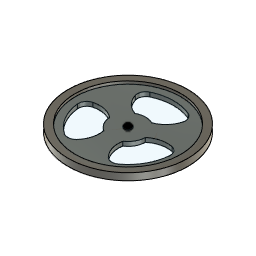
integerater v4 (Autodesk Fusion 360 archive; units mm, degrees)
design "wheel_edited"
Autodesk Fusion 360 part; units mm, degrees
note: some values were not read from the file. Chosen so that the rebuilt part matches the saved one: which bodies a step acts on; which face or edge a step refers to. Set by a fixed rule: which sketch regions a step uses.
sketch "Sketch1" plane through (0, 0, 0) normal (0, 0, 1) x (1, 0, 0)
  circle A0 centre (0, 0) radius 12.5
  circle A1 centre (0, 0) radius 37.5
  arc A2 (-17.0167, 22.1752) -> (-6.0591, 10.9333) centre (-0.423, 27.3882) ccw
  arc A3 (5.7186, 11.1152) -> (16.3238, 22.6902) centre (-0.423, 27.3882) ccw
  arc A4 (-12.4853, -0.6052) -> (-27.8122, 2.7918) centre (-23.5074, -14.0604) ccw
  arc A5 (-10.696, -25.8245) -> (-6.439, -10.714) centre (-23.5074, -14.0604) ccw
  arc A6 (27.7127, 3.6493) -> (12.4981, -0.2194) centre (23.9303, -13.3278) ccw
  arc A7 (6.7668, -10.51) -> (11.4883, -25.4819) centre (23.9303, -13.3278) ccw
  arc A8 (-32.288, -3.7057) -> (-18.5377, -26.6946) centre (0, 0) ccw
  arc A9 (19.3532, -26.1094) -> (32.3871, -2.7068) centre (0, 0) ccw
  arc A10 (12.9348, 29.8151) -> (-13.8494, 29.4015) centre (0, 0) ccw
  arc A11 (-27.8122, 2.7918) -> (-32.288, -3.7057) centre (-26.3272, -3.0216) ccw
  arc A12 (-18.5377, -26.6946) -> (-10.696, -25.8245) centre (-15.1154, -21.7664) ccw
  arc A13 (11.4883, -25.4819) -> (19.3532, -26.1094) centre (15.7803, -21.2892) ccw
  arc A14 (32.3871, -2.7068) -> (27.7127, 3.6493) centre (26.4079, -2.2071) ccw
  arc A15 (16.3238, 22.6902) -> (12.9348, 29.8151) centre (10.5468, 24.3108) ccw
  arc A16 (-13.8494, 29.4015) -> (-17.0167, 22.1752) centre (-11.2925, 23.9735) ccw
  dimension "d1" = 65
  dimension "d2" = 25
  dimension "d3" = 75
  dimension "d6" = 6
  dimension "d7" = 6
  dimension "d8" = 6
  constraint coincident A0.centre A1.centre
  constraint coincident A0 A2.end
  constraint coincident A0 A3.start
  constraint concentric A2 A3
  constraint coincident A0 A5.end
  constraint coincident A0 A4.start
  constraint concentric A4 A5
  constraint coincident A0 A6.end
  constraint coincident A0 A7.start
  constraint concentric A6 A7
  constraint concentric A8 A9
  constraint concentric A9 A10
  constraint tangent A4 A11
  constraint tangent A8 A11
  constraint tangent A8 A12
  constraint tangent A5 A12
  constraint tangent A7 A13
  constraint tangent A9 A13
  constraint equal A12 A13
  constraint tangent A9 A14
  constraint tangent A6 A14
  constraint equal A12 A14
  constraint tangent A3 A15
  constraint tangent A10 A15
  constraint equal A12 A15
  constraint tangent A2 A16
  constraint tangent A10 A16
  measures "d1" diameter of A8
  measures "d2" diameter of A0
  measures "d3" diameter of A1
  measures "d6" radius of A11
  measures "d7" radius of A12
  measures "d8" radius of A16
extrude "Extrude1" add sketch "Sketch1" along normal blind 3 contours A0 | A1
sketch "Sketch2" plane through (0, 0, 3) normal (0, 0, 1) x (-1, 0, 0)
  arc A0 (12.4853, 0.6052) -> (27.8122, -2.7918) centre (23.5074, 14.0604) ccw
  arc A1 (12.4853, 0.6052) -> (6.439, 10.714) centre (0, 0) ccw
  arc A2 (10.696, 25.8245) -> (6.439, 10.714) centre (23.5074, 14.0604) ccw
  arc A3 (18.5377, 26.6946) -> (10.696, 25.8245) centre (15.1154, 21.7664) ccw
  arc A4 (32.288, 3.7057) -> (18.5377, 26.6946) centre (0, 0) ccw
  arc A5 (27.8122, -2.7918) -> (32.288, 3.7057) centre (26.3272, 3.0216) ccw
  arc A6 (-6.7668, 10.51) -> (-11.4883, 25.4819) centre (-23.9303, 13.3278) ccw
  arc A7 (-6.7668, 10.51) -> (-12.4981, 0.2194) centre (0, 0) ccw
  arc A8 (-27.7127, -3.6493) -> (-12.4981, 0.2194) centre (-23.9303, 13.3278) ccw
  arc A9 (-32.3871, 2.7068) -> (-27.7127, -3.6493) centre (-26.4079, 2.2071) ccw
  arc A10 (-19.3532, 26.1094) -> (-32.3871, 2.7068) centre (0, 0) ccw
  arc A11 (-11.4883, 25.4819) -> (-19.3532, 26.1094) centre (-15.7803, 21.2892) ccw
  arc A12 (-5.7186, -11.1152) -> (-16.3238, -22.6902) centre (0.423, -27.3882) ccw
  arc A13 (-5.7186, -11.1152) -> (6.0591, -10.9333) centre (0, 0) ccw
  arc A14 (17.0167, -22.1752) -> (6.0591, -10.9333) centre (0.423, -27.3882) ccw
  arc A15 (13.8494, -29.4015) -> (17.0167, -22.1752) centre (11.2925, -23.9735) ccw
  arc A16 (-12.9348, -29.8151) -> (13.8494, -29.4015) centre (0, 0) ccw
  arc A17 (-16.3238, -22.6902) -> (-12.9348, -29.8151) centre (-10.5468, -24.3108) ccw
  circle A18 centre (0, 0) radius 37.5
  circle A19 centre (0, 0) radius 2.3
  line L0 (-1.5578, 1.6921) -> (-1.5578, -1.6921)
  line L1 (1.5578, -1.6921) -> (1.5578, 1.6921)
  line L2 (1.5578, 1.6921) -> (-1.5578, -1.6921) construction
  line L3 (-1.5578, 1.6921) -> (1.5578, -1.6921) construction
  dimension "d11" = 4.6
  dimension "d42" = 3.3843
  constraint concentric A1 A19
  constraint parallel L0 L1
  constraint coincident L2 A1.centre
  constraint coincident L3 A1.centre
  constraint coincident A1.centre A4.centre
  constraint coincident A19 L0.start
  measures "d11" diameter of A19
  measures "d42" distance of L0.start L0.end
extrude "Extrude2" add sketch "Sketch2" along normal blind 1.5 contours A19 L1 | A19 L0 L1 | A19 L0
sketch "Sketch3" plane through (0, 0, 0) normal (0, 0, 1) x (1, 0, 0)
  circle A0 centre (0, 0) radius 42.5
  spline S0 degree 2 poles (3.0979, -42.3869) (0, -46) (-3.0574, -42.3899) knots 0 0 0 0.819978 0.819978 0.819978 weights 1 3 1
  spline S1 degree 2 poles (8.386, -41.6644) (5.7653, -45.6373) (2.2796, -42.4388) knots 0 0 0 0.819978 0.819978 0.819978 weights 1 3 1
  spline S2 degree 2 poles (13.5418, -40.2849) (11.4397, -44.5548) (7.5806, -41.8185) knots 0 0 0 0.819978 0.819978 0.819978 weights 1 3 1
  spline S3 degree 2 poles (18.484, -38.27) (16.9337, -42.7697) (12.762, -40.5386) knots 0 0 0 0.819978 0.819978 0.819978 weights 1 3 1
  spline S4 degree 2 poles (23.1348, -35.6515) (22.1607, -40.3101) (17.7422, -38.6195) knots 0 0 0 0.819978 0.819978 0.819978 weights 1 3 1
  spline S5 degree 2 poles (27.4207, -32.4708) (27.0381, -37.2148) (22.4426, -36.0912) knots 0 0 0 0.819978 0.819978 0.819978 weights 1 3 1
  spline S6 degree 2 poles (31.2741, -28.7781) (31.4892, -33.5326) (26.7891, -32.9938) knots 0 0 0 0.819978 0.819978 0.819978 weights 1 3 1
  spline S7 degree 2 poles (34.6344, -24.6315) (35.4436, -29.3215) (30.7131, -29.3761) knots 0 0 0 0.819978 0.819978 0.819978 weights 1 3 1
  spline S8 degree 2 poles (37.4484, -20.0964) (38.8391, -24.648) (34.1527, -25.2951) knots 0 0 0 0.819978 0.819978 0.819978 weights 1 3 1
  spline S9 degree 2 poles (39.6719, -15.2444) (41.622, -19.5858) (37.0537, -20.8152) knots 0 0 0 0.819978 0.819978 0.819978 weights 1 3 1
  spline S10 degree 2 poles (41.2697, -10.152) (43.7486, -14.2148) (39.3704, -16.007) knots 0 0 0 0.819978 0.819978 0.819978 weights 1 3 1
  spline S11 degree 2 poles (42.2166, -4.8995) (45.1852, -8.6195) (41.0661, -10.9463) knots 0 0 0 0.819978 0.819978 0.819978 weights 1 3 1
  spline S12 degree 2 poles (42.4978, 0.4303) (45.9092, -2.8884) (42.1143, -5.7131) knots 0 0 0 0.819978 0.819978 0.819978 weights 1 3 1
  spline S13 degree 2 poles (42.1088, 5.7533) (45.9092, 2.8884) (42.4982, -0.3897) knots 0 0 0 0.819978 0.819978 0.819978 weights 1 3 1
  spline S14 degree 2 poles (41.0557, 10.9856) (45.1852, 8.6195) (42.2119, 4.9398) knots 0 0 0 0.819978 0.819978 0.819978 weights 1 3 1
  spline S15 degree 2 poles (39.3551, 16.0446) (43.7486, 14.2148) (41.26, 10.1914) knots 0 0 0 0.819978 0.819978 0.819978 weights 1 3 1
  spline S16 degree 2 poles (37.0338, 20.8506) (41.622, 19.5858) (39.6573, 15.2823) knots 0 0 0 0.819978 0.819978 0.819978 weights 1 3 1
  spline S17 degree 2 poles (34.1285, 25.3277) (38.8391, 24.648) (37.4292, 20.1322) knots 0 0 0 0.819978 0.819978 0.819978 weights 1 3 1
  spline S18 degree 2 poles (30.685, 29.4054) (35.4436, 29.3215) (34.6108, 24.6645) knots 0 0 0 0.819978 0.819978 0.819978 weights 1 3 1
  spline S19 degree 2 poles (26.7576, 33.0194) (31.4892, 33.5326) (31.2466, 28.8079) knots 0 0 0 0.819978 0.819978 0.819978 weights 1 3 1
  spline S20 degree 2 poles (22.4082, 36.1127) (27.0381, 37.2148) (27.3897, 32.497) knots 0 0 0 0.819978 0.819978 0.819978 weights 1 3 1
  spline S21 degree 2 poles (17.7053, 38.6364) (22.1607, 40.3101) (23.1007, 35.6736) knots 0 0 0 0.819978 0.819978 0.819978 weights 1 3 1
  spline S22 degree 2 poles (12.7233, 40.5508) (16.9337, 42.7697) (18.4475, 38.2876) knots 0 0 0 0.819978 0.819978 0.819978 weights 1 3 1
  spline S23 degree 2 poles (7.5406, 41.8257) (11.4397, 44.5548) (13.5033, 40.2978) knots 0 0 0 0.819978 0.819978 0.819978 weights 1 3 1
  spline S24 degree 2 poles (2.239, 42.441) (5.7653, 45.6373) (8.3462, 41.6724) knots 0 0 0 0.819978 0.819978 0.819978 weights 1 3 1
  spline S25 degree 2 poles (-3.0979, 42.3869) (0, 46) (3.0574, 42.3899) knots 0 0 0 0.819978 0.819978 0.819978 weights 1 3 1
  spline S26 degree 2 poles (-8.386, 41.6644) (-5.7653, 45.6373) (-2.2796, 42.4388) knots 0 0 0 0.819978 0.819978 0.819978 weights 1 3 1
  spline S27 degree 2 poles (-13.5418, 40.2849) (-11.4397, 44.5548) (-7.5806, 41.8185) knots 0 0 0 0.819978 0.819978 0.819978 weights 1 3 1
  spline S28 degree 2 poles (-18.484, 38.27) (-16.9337, 42.7697) (-12.762, 40.5386) knots 0 0 0 0.819978 0.819978 0.819978 weights 1 3 1
  spline S29 degree 2 poles (-23.1348, 35.6515) (-22.1607, 40.3101) (-17.7422, 38.6195) knots 0 0 0 0.819978 0.819978 0.819978 weights 1 3 1
  spline S30 degree 2 poles (-27.4207, 32.4708) (-27.0381, 37.2148) (-22.4426, 36.0912) knots 0 0 0 0.819978 0.819978 0.819978 weights 1 3 1
  spline S31 degree 2 poles (-31.2741, 28.7781) (-31.4892, 33.5326) (-26.7891, 32.9938) knots 0 0 0 0.819978 0.819978 0.819978 weights 1 3 1
  spline S32 degree 2 poles (-34.6344, 24.6315) (-35.4436, 29.3215) (-30.7131, 29.3761) knots 0 0 0 0.819978 0.819978 0.819978 weights 1 3 1
  spline S33 degree 2 poles (-37.4484, 20.0964) (-38.8391, 24.648) (-34.1527, 25.2951) knots 0 0 0 0.819978 0.819978 0.819978 weights 1 3 1
  spline S34 degree 2 poles (-39.6719, 15.2444) (-41.622, 19.5858) (-37.0537, 20.8152) knots 0 0 0 0.819978 0.819978 0.819978 weights 1 3 1
  spline S35 degree 2 poles (-41.2697, 10.152) (-43.7486, 14.2148) (-39.3704, 16.007) knots 0 0 0 0.819978 0.819978 0.819978 weights 1 3 1
  spline S36 degree 2 poles (-42.2166, 4.8995) (-45.1852, 8.6195) (-41.0661, 10.9463) knots 0 0 0 0.819978 0.819978 0.819978 weights 1 3 1
  spline S37 degree 2 poles (-42.4978, -0.4303) (-45.9092, 2.8884) (-42.1143, 5.7131) knots 0 0 0 0.819978 0.819978 0.819978 weights 1 3 1
  spline S38 degree 2 poles (-42.1088, -5.7533) (-45.9092, -2.8884) (-42.4982, 0.3897) knots 0 0 0 0.819978 0.819978 0.819978 weights 1 3 1
  spline S39 degree 2 poles (-41.0557, -10.9856) (-45.1852, -8.6195) (-42.2119, -4.9398) knots 0 0 0 0.819978 0.819978 0.819978 weights 1 3 1
  spline S40 degree 2 poles (-39.3551, -16.0446) (-43.7486, -14.2148) (-41.26, -10.1914) knots 0 0 0 0.819978 0.819978 0.819978 weights 1 3 1
  spline S41 degree 2 poles (-37.0338, -20.8506) (-41.622, -19.5858) (-39.6573, -15.2823) knots 0 0 0 0.819978 0.819978 0.819978 weights 1 3 1
  spline S42 degree 2 poles (-34.1285, -25.3277) (-38.8391, -24.648) (-37.4292, -20.1322) knots 0 0 0 0.819978 0.819978 0.819978 weights 1 3 1
  spline S43 degree 2 poles (-30.685, -29.4054) (-35.4436, -29.3215) (-34.6108, -24.6645) knots 0 0 0 0.819978 0.819978 0.819978 weights 1 3 1
  spline S44 degree 2 poles (-26.7576, -33.0194) (-31.4892, -33.5326) (-31.2466, -28.8079) knots 0 0 0 0.819978 0.819978 0.819978 weights 1 3 1
  spline S45 degree 2 poles (-22.4082, -36.1127) (-27.0381, -37.2148) (-27.3897, -32.497) knots 0 0 0 0.819978 0.819978 0.819978 weights 1 3 1
  spline S46 degree 2 poles (-17.7053, -38.6364) (-22.1607, -40.3101) (-23.1007, -35.6736) knots 0 0 0 0.819978 0.819978 0.819978 weights 1 3 1
  spline S47 degree 2 poles (-12.7233, -40.5508) (-16.9337, -42.7697) (-18.4475, -38.2876) knots 0 0 0 0.819978 0.819978 0.819978 weights 1 3 1
  spline S48 degree 2 poles (-7.5406, -41.8257) (-11.4397, -44.5548) (-13.5033, -40.2978) knots 0 0 0 0.819978 0.819978 0.819978 weights 1 3 1
  spline S49 degree 2 poles (-2.239, -42.441) (-5.7653, -45.6373) (-8.3462, -41.6724) knots 0 0 0 0.819978 0.819978 0.819978 weights 1 3 1
  circle A1 centre (0, 0) radius 37.5
  dimension "d17" = 85
  dimension "d22" = 360
  dimension "d23" = 75
  constraint coincident A0.centre A1.centre
  constraint coincident A0 S0.end
  constraint coincident A0 S0.start
  measures "d17" diameter of A0
  measures "d23" diameter of A1
extrude "Extrude4" add sketch "Sketch3" along normal blind 5 contours A0
extrude "Extrude5" cut 1 faces at (-0.2801, 0.7137, 4.5) along direction (0, 0, -1) blind 3
extrude "Extrude6" add 1 faces at (-0.2801, 0.7137, 1.5) along direction (0, 0, 1) blind 0.9
extrude "Extrude8" cut sketch "Sketch2" against normal blind 3 contours A19 L0 L1
extrude "Extrude7" cut sketch "Sketch2" against normal blind 3 contours A19 L0 L1

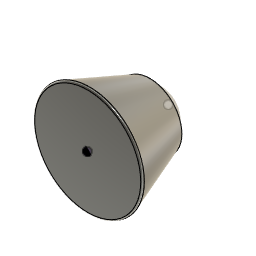
design "front_wheel v2 v3"
Autodesk Fusion 360 part; units mm, degrees
sketch "Sketch9" plane through (0, 0, 0) normal (0, 1, 0) x (1, 0, 0)
  circle A0 centre (0, 0) radius 17.5
  dimension "d12" = 35
  constraint coincident A0.centre origin
  measures "d12" diameter of A0
ref_plane "WorkPlane3" through (0, 20, 0) normal (0, 1, 0) x (0, 0, 1)
sketch "Sketch10" plane through (0, 20, 0) normal (0, 1, 0) x (1, 0, 0)
  circle A0 centre (0, 0) radius 10
  dimension "d14" = 20
  constraint coincident A0.centre origin
  measures "d14" diameter of A0
loft "Loft2" add profiles "Sketch10", "Sketch9" section 1 section 2 makes body 1
sphere "SpherePrimitive2" add diameter 19 placed x (-1, 0, 0) y (0, 0, 1) z (0, 1, 0) at (0, 20, 0) separate body makes body 2
move_body "MoveFace2" bodies 2 to x (1, 0, 0) y (0, 1, 0) z (0, 0, 1) at (0, -4, 0) on bodies 2
fillet "Fillet1" radius 0.5 1 faces at (11.6067, 4.4444, 10.7694) on bodies 1
sketch "Sketch14" plane through (0, 0, 0) normal (0, 0, 1) x (1, 0, 0)
  point P0 (0, 25.5)
  dimension "d19" = 25.5
  measures "d19" distance of origin P0

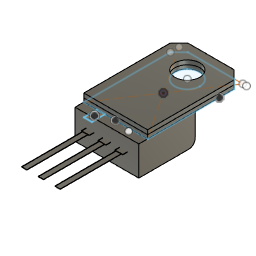
design "lm7805 v1"
Autodesk Fusion 360 part; units mm, degrees
sketch "Sketch1" plane through (0, 0, 0) normal (0, 0, 1) x (1, 0, 0)
  line L0 (4.85, -7.25) -> (-4.85, -7.25)
  line L1 (-4.85, -7.25) -> (-4.85, 5.913)
  line L2 (-3.513, 7.25) -> (3.5128, 7.25)
  line L3 (4.85, 5.9128) -> (4.85, -7.25)
  line L4 (4.85, -7.25) -> (-4.85, 7.25) construction
  line L5 (-4.85, -7.25) -> (4.85, 7.25) construction
  line L6 (-1.625, -7.2509) -> (-2.825, -7.2509)
  line L7 (-2.825, -7.2509) -> (-2.825, -9.2509)
  line L8 (-2.825, -9.2509) -> (-1.625, -9.2509)
  line L9 (-1.625, -9.2509) -> (-1.625, -7.2509)
  line L10 (-1.625, -7.2509) -> (-2.825, -9.2509) construction
  line L11 (-2.825, -7.2509) -> (-1.625, -9.2509) construction
  circle A0 centre (0, 3.65) radius 1.9
  line L12 (3.5128, 7.25) -> (4.85, 5.9128)
  line L13 (3.5128, 7.25) -> (5.4039, 7.25) construction
  line L14 (-4.8502, 5.9128) -> (-3.513, 7.25)
  point P0 (0, -7.25)
  point P1 (-2.225, -8.2509)
  point P2 (2.425, -7.6949)
  point P3 (-2.225, -8.2509)
  point P4 (4.85, 3.65)
  dimension "d1" = 9.7
  dimension "d2" = 14.5
  dimension "d3" = 1.2
  dimension "d4" = 2
  dimension "d27" = 3.6
  dimension "d28" = 3.8
  dimension "d37" = 45
  constraint horizontal L0
  constraint perpendicular L0 L1
  constraint parallel L0 L2
  constraint parallel L1 L3
  constraint coincident L4 origin
  constraint coincident L5 origin
  constraint midpoint L0 P0
  constraint horizontal L6
  constraint perpendicular L6 L7
  constraint parallel L6 L8
  constraint parallel L7 L9
  constraint coincident L10 P3
  constraint coincident L11 P3
  constraint coincident P3 P1
  constraint coincident L3 P4
  constraint horizontal L13
  constraint coincident L14 L1.end
  measures "d1" distance of L4.end L5.end
  measures "d2" distance of L0.end L4.end
  measures "d3" distance of L7.end L8.end
  measures "d4" distance of L6.end L7.end
  measures "d27" distance of L5.end P4
  measures "d28" diameter of A0
  measures "d37" angle of L12 L13
extrude "Extrude1" add sketch "Sketch1" along normal blind 0.05 contours L0 L6 L7 L8 L9 makes body 1
sketch "Sketch3" plane through (0, 0, 0.05) normal (0, 0, 1) x (-1, 0, 0)
  line L0 (1.625, 9.2509) -> (1.625, 7.2509)
  line L1 (1.625, 7.2509) -> (2.825, 7.2509)
  line L2 (2.825, 7.2509) -> (2.825, 9.2509)
  line L3 (2.825, 9.2509) -> (1.625, 9.2509)
  line L4 (2.625, 9.2509) -> (1.825, 9.2509)
  line L5 (2.625, 9.2509) -> (1.825, 9.2509)
  line L6 (1.825, 9.2509) -> (1.825, 18.5509)
  line L7 (1.825, 18.5509) -> (2.625, 18.5509)
  line L8 (2.625, 18.5509) -> (2.625, 9.2509)
  point P0 (2.225, 9.2509)
  dimension "d9" = 0.8
  dimension "d10" = 0.8
  dimension "d11" = 9.3
  constraint midpoint L3 P0
  constraint coincident L3 L4.start
  constraint perpendicular L2 L4
  constraint midpoint P0 L4
  constraint horizontal L5
  constraint vertical L6
  constraint horizontal L7
  constraint vertical L8
  measures "d9" distance of L4.start L4.end
  measures "d10" distance of L4.start L4.end
  measures "d11" distance of L4.start L7.end
extrude "Extrude3" add sketch "Sketch3" along normal blind 0.05 separate body contours L3 L4 L5 L6 L7 L8 makes body 2
move_body "Move1" bodies 2 to x (1, 0, 0) y (0, 1, 0) z (0, 0, 1) at (0, 0, -0.05)
pattern_linear "R-Pattern1" count 3 spacing 2.54 along (1, 0, 0) of bodies 1 2 makes body 3 at (0.515, -8.5839, 0) makes body 4 at (3.055, -8.5839, 0) makes body 5 at (0.1817, -12.3509, 0) makes body 6 at (2.7217, -12.3509, 0)
move_body "Move2" bodies 1 2 3 4 5 6 to x (1, 0, 0) y (0, 1, 0) z (0, 0, 1) at (-0.4, 0, 0)
extrude "Extrude4" add sketch "Sketch1" along normal blind 1.2 separate body contours L0 L1 L2 L3 L6 L12 L14 | A0 makes body 7
sketch "Sketch5" plane through (4.85, 0, 0) normal (1, 0, 0) x (0, 1, 0)
  line L0 (-7.25, 0) -> (5.9128, 0)
  line L1 (5.9128, 1.2) -> (-7.25, 1.2)
  line L2 (-7.25, 1.2) -> (-7.25, 0)
  line L3 (5.9128, 0) -> (0.0128, 0)
  line L4 (0.0128, 0) -> (-8.5872, 0)
  line L5 (-8.5872, 0) -> (-8.5872, -4.5)
  line L6 (-8.5872, -4.5) -> (0.0128, -4.5)
  line L7 (0.0128, -4.5) -> (0.0128, 0)
  line L8 (5.9128, 0) -> (5.9128, 1.2)
  dimension "d21" = 5.9
  dimension "d22" = 4.5
  constraint coincident L0.end L3.start
  constraint horizontal L4
  constraint vertical L5
  constraint horizontal L6
  constraint vertical L7
  measures "d21" distance of L0.end L3.end
  measures "d22" distance of L3.end L6.end
extrude "Extrude5" add sketch "Sketch5" against normal blind 9.7 contours L0 L4 L5 L6 L7 bodies 7
move_body "Move3" bodies 4 5 6 3 2 1 to x (1, 0, 0) y (0, 1, 0) z (0, 0, 1) at (0, 0, -2)
fillet "Fillet1" radius 1 1 edges at (0, 0.0128, -4.5) on bodies 7
extrude "Extrude2" add sketch "Sketch1" along normal blind 0.55 separate body contours L0 L1 L2 L3 L6 L12 L14 | A0 makes body 8
extrude "Extrude9" cut sketch "Sketch1" along normal blind 1.2 contours A0 bodies 7 8

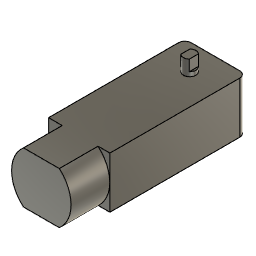
design "gear_motor_edited"
Autodesk Fusion 360 part; units mm, degrees
sketch "Sketch1" plane through (0, 0, 0) normal (0, 0, 1) x (1, 0, 0)
  line L0 (-17.7, 40) -> (0.2, 40)
  line L1 (2.5, 37.7) -> (2.5, -10)
  line L2 (2.5, -10) -> (-20, -10)
  line L3 (-20, -10) -> (-20, 37.7)
  arc A0 (-17.7, 40) -> (-20, 37.7) centre (-17.7, 37.7) ccw
  arc A1 (2.5, 37.7) -> (0.2, 40) centre (0.2, 37.7) ccw
  point P0 (-20, 40)
  point P1 (2.5, 40)
  dimension "d2" = 22.5
  dimension "d3" = 50
  dimension "d4" = 2.3
  constraint horizontal L0
  constraint vertical L1
  constraint horizontal L2
  constraint vertical L3
  constraint coincident P0 L3
  constraint coincident P0 L0
  constraint tangent L3 A0
  constraint tangent L0 A0
  constraint coincident P1 L0
  constraint coincident P1 L1
  constraint tangent L0 A1
  constraint tangent L1 A1
  constraint equal A0 A1
  measures "d2" distance of P0 P1
  measures "d3" distance of P0 L2.end
  measures "d4" radius of A0
extrude "Extrude1" add sketch "Sketch1" along normal blind 18.8
sketch "Sketch2" plane through (0, -10, 0) normal (0, -1, 0) x (1, 0, 0)
  line L0 (-20, 0) -> (2.5, 0)
  line L1 (2.5, 0) -> (2.5, 18.8)
  line L2 (2.5, 18.8) -> (-20, 18.8)
  line L3 (-20, 18.8) -> (-20, 0)
  line L4 (-15.0101, 18.8) -> (-2, 18.8)
  line L5 (-2, 0) -> (-15.0101, 0)
  arc A0 (-1.8591, 0) -> (-1.8591, 18.8) centre (-9.9731, 9.4) ccw
  arc A1 (-15.013, 18.8) -> (-15.013, 0) centre (-7.0677, 9.4) ccw
  constraint horizontal L4
  constraint horizontal L5
  constraint coincident L0 L5.start
  constraint coincident L2 L4.start
  constraint coincident L2 A1.start
  constraint coincident L2 A0.end
  constraint coincident L0 A0.start
  constraint coincident L0 A1.end
extrude "Extrude2" add sketch "Sketch2" along normal blind 14.2 contours L0 L2 L4 L5 A0 A1
sketch "Sketch3" plane through (0, 0, 18.8) normal (0, 0, 1) x (-1, 0, 0)
  line L0 (-2.5, 10) -> (-2.5, -37.7)
  arc A0 (-2.5, -37.7) -> (-0.2, -40) centre (-0.2, -37.7) ccw
  line L1 (-0.2, -40) -> (17.7, -40)
  arc A1 (17.7, -40) -> (20, -37.7) centre (17.7, -37.7) ccw
  line L2 (20, -37.7) -> (20, 10)
  line L3 (20, 10) -> (15.013, 10)
  line L4 (15.013, 10) -> (15.013, 24.2)
  line L5 (15.013, 24.2) -> (1.8591, 24.2)
  line L6 (1.8591, 24.2) -> (1.8591, 10)
  line L7 (1.8591, 10) -> (-2.5, 10)
  circle A2 centre (8.75, -30.5159) radius 2.3
  dimension "d9" = 22.5
  dimension "d10" = 4.6
  measures "d9" distance of L0 L2
  measures "d10" diameter of A2
extrude "Extrude3" add sketch "Sketch3" along normal blind 1.6 contours A2
sketch "Sketch4" plane through (0, 0, 20.4) normal (0, 0, 1) x (-1, 0, 0)
  circle A0 centre (8.75, -30.5159) radius 2.3
  line L0 (7.5216, -28.6683) -> (7.5284, -28.6683)
  line L1 (9.9779, -28.6683) -> (9.9848, -28.6683)
  line L2 (9.9848, -32.2683) -> (9.9428, -32.2683)
  line L3 (7.5635, -32.2683) -> (7.5216, -32.2683)
  line L4 (10.3078, -28.8238) -> (10.3078, -32.208)
  line L5 (7.1922, -32.208) -> (7.1922, -28.8238)
  line L6 (7.1922, -28.8238) -> (10.3078, -32.208) construction
  line L7 (10.3078, -28.8238) -> (7.1922, -32.208) construction
  point P0 (8.75, -30.5159)
  dimension "d13" = 3.6
  constraint horizontal L2
  constraint horizontal L0
  constraint collinear L0 L1
  constraint collinear L2 L3
  constraint parallel L4 L5
  constraint coincident L6 P0
  constraint coincident L7 P0
  constraint coincident A0 L5.end
  constraint coincident P0 A0.centre
  measures "d13" distance of L2.start L1.end
extrude "Extrude9" add sketch "Sketch4" along normal blind 4 contours A0 L4 L5
sketch "Sketch6" plane through (0, 0, 0) normal (1, 0, 0) x (0, 1, 0)
  line L0 (-17.9523, 18.8565) -> (-17.9523, 21.2632)
  line L1 (-17.9523, 21.2632) -> (-22.9523, 21.2632)
  line L2 (-22.9523, 21.2632) -> (-22.9523, 20.2632)
  line L3 (-22.9523, 20.2632) -> (-18.9025, 20.2632)
  line L4 (-18.9025, 20.2632) -> (-18.9025, 18.8565)
  line L5 (-18.9025, 18.8565) -> (-17.9523, 18.8565)
  dimension "d17" = 5
  constraint vertical L0
  constraint perpendicular L0 L1
  constraint perpendicular L1 L2
  constraint perpendicular L2 L3
  constraint perpendicular L3 L4
  constraint perpendicular L0 L5
  measures "d17" distance of L0.end L1.end
extrude "Extrude5" [suppressed]
move_body "Move1" [suppressed]
move_body "Move2" [suppressed]
sketch "Sketch7" plane through (0, 0, 21.2632) normal (0, 0, 1) x (-1, 0, 0)
  line L0 (5, 18.9523) -> (5, 23.9523)
  line L1 (5, 23.9523) -> (2, 23.9523)
  line L2 (2, 23.9523) -> (2, 18.9523)
  line L3 (2, 18.9523) -> (5, 18.9523)
  circle A0 centre (3.5, 22.7587) radius 0.75
  dimension "d20" = 1.5
  measures "d20" diameter of A0
extrude "Extrude6" [suppressed]
copy_body "CopyPasteBodies2" [suppressed]
move_body "Move4" [suppressed]
move_body "Move5" [suppressed]
move_body "Move6" [suppressed]
move_body "Move7" [suppressed]
sketch "Sketch8" plane through (0, -24.2, 0) normal (0, -1, 0) x (1, 0, 0)
  line L0 (-1.8591, 18.8) -> (-15.013, 18.8)
  arc A0 (-15.013, 18.8) -> (-15.013, 0) centre (-7.0677, 9.4) ccw
  line L1 (-15.013, 0) -> (-1.8591, 0)
  arc A1 (-1.8591, 0) -> (-1.8591, 18.8) centre (-9.9731, 9.4) ccw
  line L2 (-8.4361, 0) -> (-8.4361, 18.8) construction
  circle A2 centre (-8.4361, 9.4) radius 3
  circle A3 centre (-8.4361, 9.4) radius 1
  dimension "d23" = 6
  dimension "d24" = -2
  constraint midpoint L1 L2.start
  constraint midpoint L0 L2.end
  constraint midpoint L2 A2.centre
  measures "d23" diameter of A2
extrude "Extrude7" [suppressed]
extrude "Extrude8" [suppressed]

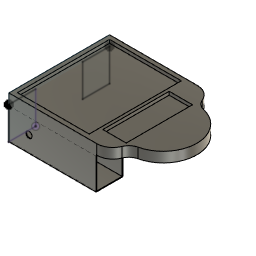
design "chassis_edited"
Autodesk Fusion 360 part; units mm, degrees
sketch "Sketch1" plane through (0, 0, 0) normal (0, 0, 1) x (1, 0, 0)
  line L0 (-100, 50) -> (-22.5, 50)
  line L1 (-22.5, -25) -> (-100, -25)
  line L2 (-100, -25) -> (-100, 50)
  arc A0 (-22.5, -12.5) -> (-22.5, 37.5) centre (-22.5, 12.5) ccw
  line L3 (-22.5, 50) -> (-22.5, 37.5)
  line L4 (-22.5, -12.5) -> (-22.5, -25)
  line L5 (-22.5, 37.5) -> (-22.5, -12.5) construction
  point P0 (-22.5, 12.5)
  dimension "d1" = 77.5
  dimension "d2" = 75
  dimension "d3" = 25
  dimension "d4" = 12.5
  constraint horizontal L0
  constraint vertical L3
  constraint horizontal L1
  constraint vertical L2
  constraint coincident A0.start L3
  constraint collinear L3 L4
  constraint coincident P0 L3
  constraint coincident P0 A0.centre
  measures "d1" distance of L0.start L0.end
  measures "d2" distance of L0.start L1.end
  measures "d3" radius of A0
  measures "d4" distance of L0.end A0.end
extrude "Extrude1" add sketch "Sketch1" along normal blind 5
extrude "Extrude2" add 1 faces at (-74.1667, 4.1667, 5) along direction (0, 0, 1) blind 2.5
fillet "Fillet1" radius 12 1 edges at (-22.5, 50, 3.75)
fillet "Fillet2" radius 12 1 edges at (-22.5, -25, 3.75)
fillet "Fillet3" radius 9 1 edges at (-22.5, -12.5, 3.75)
fillet "Fillet4" radius 9 1 edges at (-22.5, 37.5, 3.75)
sketch "Sketch2" plane through (0, 0, 7.5) normal (0, 0, 1) x (-1, 0, 0)
  arc A0 (16.9432, 11.8746) -> (16.9432, -36.8746) centre (22.5, -12.5) ccw
  arc A1 (23.3244, -42.3711) -> (16.9432, -36.8746) centre (14.9428, -45.6495) ccw
  arc A2 (23.3244, -42.3711) -> (34.5, -50) centre (34.5, -38) ccw
  line L0 (34.5, -50) -> (100, -50)
  line L1 (100, -50) -> (100, 25)
  line L2 (100, 25) -> (34.5, 25)
  arc A3 (34.5, 25) -> (23.3244, 17.3711) centre (34.5, 13) ccw
  arc A4 (16.9432, 11.8746) -> (23.3244, 17.3711) centre (14.9428, 20.6495) ccw
  line L3 (97, -47) -> (43.585, -47)
  line L4 (43.585, -47) -> (43.585, 21.615)
  line L5 (43.585, 21.615) -> (97, 21.615)
  line L6 (97, 21.615) -> (97, -47)
  dimension "d17" = 53.415
  dimension "d18" = 68.615
  constraint horizontal L3
  constraint vertical L4
  constraint horizontal L5
  constraint vertical L6
  measures "d17" distance of L3.start L3.end
  measures "d18" distance of L3.start L5.end
extrude "Extrude3" cut sketch "Sketch2" against normal blind 2.5 contours L3 L4 L5 L6
sketch "Sketch3" plane through (0, 0, 7.5) normal (0, 0, 1) x (-1, 0, 0)
  line L0 (43.585, -47) -> (43.585, 21.615)
  line L1 (43.585, 21.615) -> (97, 21.615)
  line L2 (97, 21.615) -> (97, -47)
  line L3 (97, -47) -> (43.585, -47)
  arc A0 (16.9432, 11.8746) -> (16.9432, -36.8746) centre (22.5, -12.5) ccw
  arc A1 (23.3244, -42.3711) -> (16.9432, -36.8746) centre (14.9428, -45.6495) ccw
  arc A2 (23.3244, -42.3711) -> (34.5, -50) centre (34.5, -38) ccw
  line L4 (34.5, -50) -> (100, -50)
  line L5 (100, -50) -> (100, 25)
  line L6 (100, 25) -> (34.5, 25)
  arc A3 (34.5, 25) -> (23.3244, 17.3711) centre (34.5, 13) ccw
  arc A4 (16.9432, 11.8746) -> (23.3244, 17.3711) centre (14.9428, 20.6495) ccw
  dimension "d21" = 75
  measures "d21" distance of L4.end L5.end
sketch "Sketch4" plane through (0, 0, 7.5) normal (0, 0, 1) x (-1, 0, 0)
  line L0 (43.585, -47) -> (43.585, 21.615)
  line L1 (43.585, 21.615) -> (97, 21.615)
  line L2 (97, 21.615) -> (97, -47)
  line L3 (97, -47) -> (43.585, -47)
  arc A0 (16.9432, 11.8746) -> (16.9432, -36.8746) centre (22.5, -12.5) ccw
  arc A1 (23.3244, -42.3711) -> (16.9432, -36.8746) centre (14.9428, -45.6495) ccw
  arc A2 (23.3244, -42.3711) -> (34.5, -50) centre (34.5, -38) ccw
  line L4 (34.5, -50) -> (100, -50)
  line L5 (100, -50) -> (100, 25)
  line L6 (100, 25) -> (34.5, 25)
  arc A3 (34.5, 25) -> (23.3244, 17.3711) centre (34.5, 13) ccw
  arc A4 (16.9432, 11.8746) -> (23.3244, 17.3711) centre (14.9428, 20.6495) ccw
  line L7 (41.3608, 13.6241) -> (41.3608, -35.7367)
  line L8 (41.3608, -35.7367) -> (23.985, -35.7367)
  line L9 (23.985, -35.7367) -> (23.985, 13.6241)
  line L10 (23.985, 13.6241) -> (41.3608, 13.6241)
extrude "Extrude5" cut sketch "Sketch4" against normal blind 2.5 contours L7 L8 L9 L10
sketch "Sketch6" plane through (-100, 0, 0) normal (-1, 0, 0) x (0, -1, 0)
  line L0 (-50, 0) -> (25, 0)
  line L1 (25, 0) -> (25, 7.5)
  line L2 (25, 7.5) -> (-50, 7.5)
  line L3 (-50, 7.5) -> (-50, 0)
  line L4 (25, 0) -> (5, 0)
  line L5 (5, 0) -> (5, -24)
  line L6 (5, -24) -> (25, -24)
  line L7 (25, -24) -> (25, 0)
  dimension "d30" = 20
  dimension "d31" = 24
  constraint horizontal L4
  constraint vertical L5
  constraint horizontal L6
  constraint vertical L7
  constraint coincident L0.end L1.start
  measures "d30" distance of L0.end L4.end
  measures "d31" distance of L0.end L6.end
extrude "Extrude12" add sketch "Sketch6" against normal blind 65 contours L0 L4 L5 L6 L7
sketch "Sketch7" plane through (-100, 0, 0) normal (-1, 0, 0) x (0, -1, 0)
  line L0 (25, -24) -> (25, 7.5)
  line L1 (25, 7.5) -> (-50, 7.5)
  line L2 (-50, 7.5) -> (-50, 0)
  line L3 (-50, 0) -> (5, 0)
  line L4 (-50, 0) -> (-30, 0)
  line L5 (-30, 0) -> (-30, -24)
  line L6 (-30, -24) -> (-50, -24)
  line L7 (-50, -24) -> (-50, 0)
  line L8 (5, 0) -> (5, -24)
  line L9 (5, -24) -> (25, -24)
  dimension "d35" = 24
  dimension "d38" = 20
  constraint horizontal L4
  constraint vertical L5
  constraint horizontal L6
  constraint vertical L7
  constraint coincident L2.end L3.start
  measures "d35" distance of L2.end L6.end
  measures "d38" distance of L2.end L4.end
extrude "Extrude13" add sketch "Sketch7" against normal blind 65 contours L3 L4 L5 L6 L7
sketch "Sketch13" plane through (-100, 40, -12) normal (-1, 0, 0) x (0, -1, 0)
  line L0 (-9.5, -11.5) -> (9.3, -11.5)
  line L1 (9.3, -11.5) -> (9.3, 11)
  line L2 (9.3, 11) -> (-9.5, 11)
  line L3 (-9.5, 11) -> (-9.5, -11.5)
  line L4 (10, -12) -> (-10, -12)
  line L5 (-10, -12) -> (-10, 12)
  dimension "d60" = 18.8
  dimension "d61" = 22.5
  dimension "d66" = 0.5
  dimension "d67" = 0.5
  constraint horizontal L0
  constraint vertical L1
  constraint horizontal L2
  constraint vertical L3
  measures "d60" distance of L0.start L0.end
  measures "d61" distance of L0.start L2.end
  measures "d66" distance of L0.start L4
  measures "d67" distance of L0.start L5
extrude "Extrude15" cut sketch "Sketch13" against normal blind 70
sketch "Sketch14" plane through (-100, -15, -12) normal (-1, 0, 0) x (0, -1, 0)
  line L0 (9.5, -11.5) -> (-9.3, -11.5)
  line L1 (-9.3, -11.5) -> (-9.3, 11)
  line L2 (-9.3, 11) -> (9.5, 11)
  line L3 (9.5, 11) -> (9.5, -11.5)
  line L4 (10, -12) -> (10, 12)
  line L5 (-10, -12) -> (10, -12)
  dimension "d68" = 18.8
  dimension "d69" = 22.5
  dimension "d70" = 0.5
  dimension "d71" = 0.5
  constraint horizontal L0
  constraint vertical L1
  constraint horizontal L2
  constraint vertical L3
  measures "d68" distance of L0.start L0.end
  measures "d69" distance of L0.start L2.end
  measures "d70" distance of L0.start L4
  measures "d71" distance of L0.start L5
extrude "Extrude19" cut sketch "Sketch14" against normal blind 69
sketch "Sketch18" plane through (0, -25, 0) normal (0, -1, 0) x (1, 0, 0)
  line L0 (-34.5, 0) -> (-34.5, 7.5)
  line L1 (-34.5, 7.5) -> (-100, 7.5)
  line L2 (-100, 7.5) -> (-100, -24)
  line L3 (-100, -24) -> (-35, -24)
  line L4 (-35, -24) -> (-35, 0)
  line L5 (-35, 0) -> (-34.5, 0)
  line L6 (-85, 0) -> (-85, -24) construction
  circle A0 centre (-85, -12) radius 2.3
  point P0 (-100, -24)
  dimension "d83" = 4.6
  dimension "d84" = 15
  constraint coincident L3 L6.end
  constraint perpendicular L3 L6
  constraint midpoint L6 A0.centre
  measures "d83" diameter of A0
  measures "d84" distance of L6.end P0
extrude "Extrude22" cut sketch "Sketch18" against normal blind 1 contours A0
sketch "Sketch19" plane through (0, 50, 0) normal (0, 1, 0) x (-1, 0, 0)
  line L0 (34.5, 7.5) -> (34.5, 0)
  line L1 (34.5, 0) -> (35, 0)
  line L2 (35, 0) -> (35, -24)
  line L3 (35, -24) -> (100, -24)
  line L4 (100, -24) -> (100, 7.5)
  line L5 (100, 7.5) -> (34.5, 7.5)
  line L6 (85, 0) -> (85, -24) construction
  circle A0 centre (85, -12) radius 2.3
  dimension "d87" = 4.6
  dimension "d88" = 15
  constraint coincident L3 L6.end
  constraint perpendicular L3 L6
  constraint midpoint L6 A0.centre
  measures "d87" diameter of A0
  measures "d88" distance of L3.end L6.end
extrude "Extrude23" cut sketch "Sketch19" against normal blind 1 contours A0
extrude "Extrude25" [suppressed]

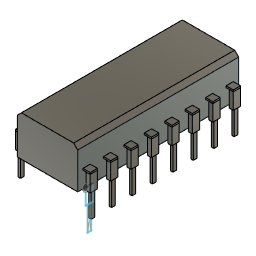
design "ic_l293d v1"
Autodesk Fusion 360 part; units mm, degrees
sketch "Sketch1" plane through (0, 0, 0) normal (0, 0, 1) x (1, 0, 0)
  line L0 (3.75, -10) -> (-3.75, -10)
  line L1 (-3.75, -10) -> (-3.75, 10)
  line L2 (-3.75, 10) -> (3.75, 10)
  line L3 (3.75, 10) -> (3.75, -10)
  line L4 (3.75, -10) -> (-3.75, 10) construction
  line L5 (-3.75, -10) -> (3.75, 10) construction
  dimension "d1" = 7.5
  dimension "d2" = 20
  constraint horizontal L0
  constraint perpendicular L0 L1
  constraint parallel L0 L2
  constraint parallel L1 L3
  constraint coincident L4 origin
  constraint coincident L5 origin
  measures "d1" distance of L1.end L2.end
  measures "d2" distance of L0.end L1.end
extrude "Extrude1" add sketch "Sketch1" along normal blind 5 makes body 1
chamfer "Chamfer1" distance 0.5 angle 45 1 edges at (3.75, 0, 5) on bodies 1
chamfer "Chamfer2" distance 0.5 angle 45 1 edges at (-3.75, 0, 5) on bodies 1
sketch "Sketch3" plane through (3.75, 0, 0) normal (1, 0, 0) x (0, 1, 0)
  line L0 (10, 4.5) -> (-10, 4.5)
  line L1 (-10, 4.5) -> (-10, 0)
  line L2 (-10, 0) -> (10, 0)
  line L3 (10, 0) -> (10, 4.5)
  line L4 (-9, 0) -> (-8.1, 0)
  line L5 (-8.1, 0) -> (-8.1, -2)
  line L6 (-8.1, -2) -> (-9, -2)
  line L7 (-9, -2) -> (-9, 0)
  line L8 (-8.325, -5) -> (-8.775, -5)
  line L9 (-8.775, -5) -> (-8.775, -2)
  line L10 (-8.775, -2) -> (-8.325, -2)
  line L11 (-8.325, -2) -> (-8.325, -5)
  line L12 (-8.325, -5) -> (-8.775, -2) construction
  line L13 (-8.775, -5) -> (-8.325, -2) construction
  dimension "d7" = 0.9
  dimension "d8" = 2
  dimension "d9" = 0.45
  dimension "d10" = 3
  constraint horizontal L4
  constraint vertical L5
  constraint vertical L7
  constraint coincident L2 L4.start
  constraint horizontal L8
  constraint perpendicular L8 L9
  constraint parallel L8 L10
  constraint parallel L9 L11
  measures "d7" distance of L4.start L4.end
  measures "d8" distance of L4.start L6.end
  measures "d9" distance of L9.end L10.end
  measures "d10" distance of L8.end L9.end
extrude "Extrude2" add sketch "Sketch3" along normal blind 0.5 separate body contours L2 L4 L5 L6 L7 L10 makes body 2
extrude "Extrude3" add sketch "Sketch3" along normal blind 0.3 separate body contours L6 L8 L9 L10 L11 makes body 3
move_body "Move1" bodies 3 to x (1, 0, 0) y (0, 1, 0) z (0, 0, 1) at (0.1, 0, 0)
move_body "Move2" bodies 2 3 to x (1, 0, 0) y (0, 1, 0) z (0, 0, 1) at (0.4, 0, 2)
sketch "Sketch4" plane through (0, 0, 2) normal (0, 0, 1) x (-1, 0, 0)
  line L0 (-4.15, 8.1) -> (-4.15, 9)
  line L1 (-4.15, 9) -> (-4.65, 9)
  line L2 (-4.65, 9) -> (-4.65, 8.1)
  line L3 (-4.65, 8.1) -> (-4.15, 8.1)
  line L4 (-4.65, 9) -> (-4.65, 8.1)
  line L5 (-3.75, 8.1) -> (-4.65, 8.1)
  line L6 (-3.75, 8.1) -> (-3.75, 9)
  line L7 (-3.75, 9) -> (-4.65, 9)
  constraint coincident L1.end L2.start
  constraint coincident L2.end L3.start
  constraint perpendicular L4 L5
  constraint perpendicular L5 L6
extrude "Extrude4" add sketch "Sketch4" along normal blind 0.2 separate body makes body 4
pattern_linear "R-Pattern1" count 8 spacing 2.54 along (0, 1, 0) of bodies 2 3 4 makes body 5 at (4.15, -5.935, 1.3333) makes body 6 at (4.15, -3.395, 1.3333) makes body 7 at (4.15, -0.855, 1.3333) makes body 8 at (4.15, 1.685, 1.3333) makes body 9 at (4.15, 4.225, 1.3333) makes body 10 at (4.15, 6.765, 1.3333) makes body 11 at (4.15, 9.305, 1.3333) makes body 12 at (4.25, -6.085, -1) makes body 13 at (4.25, -3.545, -1) makes body 14 at (4.25, -1.005, -1) makes body 15 at (4.25, 1.535, -1) makes body 16 at (4.25, 4.075, -1) makes body 17 at (4.25, 6.615, -1) makes body 18 at (4.25, 9.155, -1) makes body 19 at (4.3167, -5.86, 2.2) makes body 20 at (4.3167, -3.32, 2.2) makes body 21 at (4.3167, -0.78, 2.2) makes body 22 at (4.3167, 1.76, 2.2) makes body 23 at (4.3167, 4.3, 2.2) makes body 24 at (4.3167, 6.84, 2.2) makes body 25 at (4.3167, 9.38, 2.2)
move_body "Move3" bodies 2 19 20 11 12 10 9 8 3 16 15 13 14 4 25 24 23 22 21 17 18 6 7 5 to x (1, 0, 0) y (0, 1, 0) z (0, 0, 1) at (0, -0.35, 0)
copy_body "CopyPasteBodies1" bodies 2 3 4 5 6 7 8 9 10 11 12 13 14 15 16 17 18 19 20 21 22 23 24 25 makes body 26 makes body 27 makes body 28 makes body 29 makes body 30 makes body 31 makes body 32 makes body 33 makes body 34 makes body 35 makes body 36 makes body 37 makes body 38 makes body 39 makes body 40 makes body 41 makes body 42 makes body 43 makes body 44 makes body 45 makes body 46 makes body 47 makes body 48 makes body 49
move_body "Move4" bodies 26 27 28 29 30 31 32 33 34 35 36 37 38 39 40 41 42 43 44 45 46 47 48 49 to x (-1, 0, 0) y (0, -1, 0) z (0, 0, 1) at (0, 0, 0)

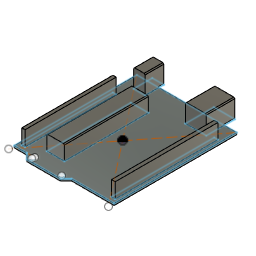
design "arduino v1"
Autodesk Fusion 360 part; units mm, degrees
sketch "Sketch1" plane through (0, 0, 0) normal (0, 0, 1) x (1, 0, 0)
  line L0 (26.7075, 34.3075) -> (-26.7075, 34.3075)
  line L1 (-26.7075, 34.3075) -> (-26.7075, -31.3075)
  line L2 (-17.0004, -34.3075) -> (0.9996, -34.3075)
  line L3 (26.7075, -31.3075) -> (26.7075, 34.3075)
  line L4 (26.7075, 34.3075) -> (-26.7075, -34.3075) construction
  line L5 (-26.7075, 34.3075) -> (26.7075, -34.3075) construction
  line L6 (-20.0004, -31.3075) -> (-17.0004, -34.3075)
  line L7 (-20.0004, -31.3075) -> (-15.7577, -31.3075) construction
  line L8 (0.9996, -34.3075) -> (3.9996, -31.3075)
  line L9 (-26.7075, -31.3075) -> (-20.0004, -31.3075)
  line L10 (3.9996, -31.3075) -> (26.7075, -31.3075)
  line L11 (-25, 19.7356) -> (-23.2405, 19.7356)
  line L12 (-23.2405, 19.7356) -> (-23.2405, -29)
  line L13 (-23.2405, -29) -> (-25, -29)
  line L14 (-25, -29) -> (-25, 19.7356)
  line L15 (23, -29) -> (23, 26)
  line L16 (25, 26) -> (25, -29)
  line L17 (23, 26) -> (25, 26)
  line L18 (25, -29) -> (23, -29)
  line L19 (8.8362, 40) -> (20, 40)
  line L20 (20, 40) -> (20, 24.762)
  line L21 (20, 24.762) -> (8.8362, 24.762)
  line L22 (8.8362, 24.762) -> (8.8362, 40)
  line L23 (-21.1638, 37) -> (-15, 37)
  line L24 (-15, 37) -> (-15, 27)
  line L25 (-15, 27) -> (-21.1638, 27)
  line L26 (-21.1638, 27) -> (-21.1638, 37)
  line L27 (-15.4468, 19.8424) -> (-6.1117, 19.8424)
  line L28 (-6.1117, 19.8424) -> (-6.1117, -25.0987)
  line L29 (-6.1117, -25.0987) -> (-15.4468, -25.0987)
  line L30 (-15.4468, -25.0987) -> (-15.4468, 19.8424)
  circle A0 centre (-16.0725, -32.5657) radius 1.05
  circle A1 centre (-0.0725, -32.5657) radius 1.05
  dimension "d1" = 53.415
  dimension "d2" = 68.615
  dimension "d3" = 3
  dimension "d4" = 45
  dimension "d24" = 2.1
  dimension "d25" = 2.1
  constraint horizontal L0
  constraint perpendicular L0 L1
  constraint parallel L0 L2
  constraint parallel L1 L3
  constraint coincident L4 origin
  constraint coincident L5 origin
  constraint perpendicular L3 L9
  constraint horizontal L7
  constraint collinear L9 L10
  constraint horizontal L11
  constraint vertical L12
  constraint horizontal L13
  constraint vertical L14
  constraint horizontal L17
  constraint vertical L16
  constraint horizontal L18
  constraint vertical L15
  constraint horizontal L19
  constraint vertical L20
  constraint horizontal L21
  constraint vertical L22
  constraint horizontal L23
  constraint vertical L24
  constraint horizontal L25
  constraint vertical L26
  constraint horizontal L27
  constraint vertical L28
  constraint horizontal L29
  constraint vertical L30
  constraint coincident L5 L27.start
  measures "d1" distance of L4.end L5.end
  measures "d2" distance of L0.end L4.end
  measures "d3" distance of L4.end L1.end
  measures "d4" angle of L6 L7
  measures "d24" diameter of A0
  measures "d25" diameter of A1
extrude "Extrude1" add sketch "Sketch1" against normal blind 1 contours L0 L1 L2 L3 L6 L8 L9 L10 L20 L21 L22 L24 L25 L26 | L0 L20 L21 L22 | L0 L24 L25 L26 | L11 L12 L13 L14 | L15 L16 L17 L18 | L27 L28 L29 L30 | A0 | A1
extrude "Extrude2" add sketch "Sketch1" along normal blind 8 contours L11 L12 L13 L14
extrude "Extrude3" add sketch "Sketch1" along normal blind 8 contours L15 L16 L17 L18
extrude "Extrude4" add sketch "Sketch1" along normal blind 10 contours L0 L20 L21 L22 | L0 L19 L20 L22
extrude "Extrude5" add sketch "Sketch1" along normal blind 10 contours L0 L24 L25 L26 | L0 L23 L24 L26
sketch "Sketch2" plane through (0, 40, 0) normal (0, 1, 0) x (-1, 0, 0)
  line L0 (-20, 0) -> (-8.8362, 0)
  line L1 (-8.8362, 0) -> (-8.8362, 10)
  line L2 (-8.8362, 10) -> (-20, 10)
  line L3 (-20, 10) -> (-20, 0)
  line L4 (-18.846, 1.154) -> (-9.9903, 1.154)
  line L5 (-9.9903, 1.154) -> (-9.9903, 8.846)
  line L6 (-9.9903, 8.846) -> (-18.846, 8.846)
  line L7 (-18.846, 8.846) -> (-18.846, 1.154)
  circle A0 centre (18, 5) radius 2.2361
  dimension "d15" = -1.154
extrude "Extrude6" cut sketch "Sketch2" against normal blind 13 contours L4 L5 L6 L7
extrude "Extrude7" cut sketch "Sketch2" against normal blind 11 contours A0
extrude "Extrude8" add sketch "Sketch1" along normal blind 8 contours L27 L28 L29 L30
chamfer "Chamfer1" distance 0.5 angle 45 6 edges at (-15.4468, -2.6281, 8) (-6.1117, -2.6281, 8) (8.8362, 32.381, 10) (20, 32.381, 10) (-15, 32, 10) (-21.1638, 32, 10)
chamfer "Chamfer2" distance 0.5 angle 45 4 edges at (8.8362, 37.1538, 0) (20, 37.1538, 0) (-21.1638, 35.6538, 0) (-15, 35.6538, 0)
extrude "Extrude9" cut sketch "Sketch1" against normal blind 1 contours A0 | A1
